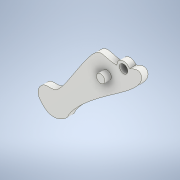
# Autodesk Inventor part: Component36
Saved by Autodesk Inventor 2022 (Build 260153000, 153)
## iProperties
Created: 2022-01-29
Part Number: Component36
Material: Generic
Document SubType Name: Modeling
Designer: Administrator
Density: 1 g/cm^3
Appearance: Default
Title: Component36
Author: Administrator
Autodesk Inventor part; units mm, degrees
ref_plane "YZ Plane" through (0, 0, 0) normal (1, 0, 0) x (0, 1, 0)
ref_plane "XZ Plane" through (0, 0, 0) normal (0, 1, 0) x (-1, 0, 0)
ref_plane "XY Plane" through (0, 0, 0) normal (0, 0, 1) x (1, 0, 0)
sketch "Sketch2" plane through (0, 0, 0) normal (0, 0, 1) x (1, 0, 0)
  circle A0 centre (18.1569, 16.7099) radius 3.25
  circle A1 centre (31.0175, 27.1749) radius 3.25
  spline S0 degree 5 poles (35.6155, 29.6037) (36.3156, 29.911) (37.8173, 30.5849) (39.9595, 31.5138) (42.4347, 32.111) (44.7655, 30.7696) (45.522, 27.5666) (43.8839, 23.4573) (39.7861, 18.7075) (33.4771, 13.4925) (25.53, 7.8047) (16.7103, 1.6544) (7.881, -4.9033) (-0.0496, -11.5568) (-6.3349, -17.8595) (-10.2076, -22.6076) (-11.7327, -25.1474) (-12.102, -26.3799) (-12.6784, -27.4169) (-14.4405, -29.0232) (-17.4072, -30.9083) (-21.1117, -32.3552) (-24.8917, -32.5969) (-28.3059, -31.3724) (-31.2897, -29.1082) (-33.7495, -26.324) (-35.5373, -23.5299) (-35.7005, -20.219) (-34.1546, -16.8547) (-31.5314, -14.4612) (-28.577, -13.7288) (-25.649, -14.0951) (-22.6659, -14.0184) (-19.3956, -11.9964) (-15.6218, -7.3504) (-11.3935, -1.1526) (-6.8872, 5.8137) (-2.3556, 12.7315) (1.9343, 18.9327) (5.7602, 23.8824) (8.3546, 26.5758) (10.0594, 27.8399) (11.1245, 28.3723) (11.646, 28.5669) (12.1676, 28.7614) (13.1888, 29.0071) (14.6963, 28.981) (16.883, 28.3621) (19.8122, 27.5131) (22.5587, 27.0894) (24.5922, 27.0161) (25.6958, 27.0472) (25.819, 27.0515) knots 0.137303 0.137303 0.137303 0.137303 0.137303 0.137303 0.155556 0.177778 0.2 0.222222 0.244444 0.266667 0.288889 0.311111 0.333333 0.355556 0.377778 0.4 0.422222 0.444444 0.466667 0.488889 0.511111 0.533333 0.555556 0.577778 0.6 0.622222 0.644444 0.666667 0.688889 0.711111 0.733333 0.755556 0.777778 0.8 0.822222 0.844444 0.866667 0.888889 0.911111 0.933333 0.955556 0.977778 1 1 1 1 1 1.022222 1.044444 1.066667 1.088889 1.091674 1.091674 1.091674 1.091674 1.091674 1.091674 weights 1 1 1 1 1 1 1 1 1 1 1 1 1 1 1 1 1 1 1 1 1 1 1 1 1 1 1 1 1 1 1 1 1 1 1 1 1 1 1 1 1 1 1 1 1 1 1 1 1 1 1 1 1
  arc A2 (35.6155, 29.6037) -> (25.819, 27.0515) centre (31.0175, 27.1749) ccw
  point P0 (0, 0)
  dimension "d4" = 6.5
  constraints: 3 centre point, 2 point on circle, 1 equal radius, 2 other
  measures "d4" diameter of A1
extrude "Extrusion1" add sketch "Sketch2" against normal blind 5 contours A0 | S0 A2
extrude "Extrusion2" add sketch "Sketch2" along normal blind 5 contours A0
equation "\"d4\" = R"
equation "\"d0\" = thickness"
equation "\"d2\" = thickness"
equation "\"R\" = 6.5"
equation "\"thickness\" = 5"
equation "\"width\" = 6.5"
equation "\"R1\" = 9"
body "Solid1"
